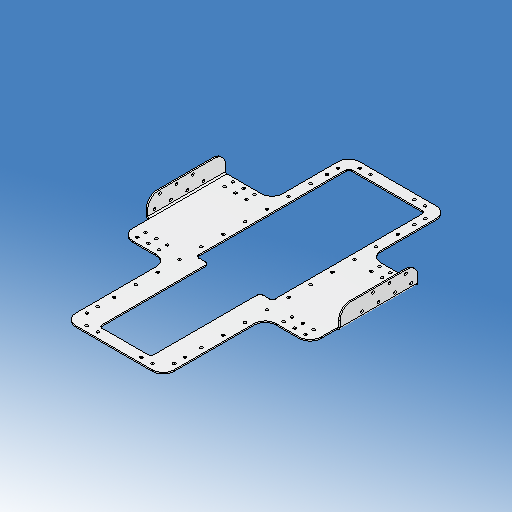
# Autodesk Inventor part: Centerpiece_bottomPlate
Saved by Autodesk Inventor 2025 (Build 290162000, 162)
## iProperties
Created: 2022-10-10
Part Number: Centerpiece_bottomPlate
Material: Aluminum 6061
Document SubType Name: Sheet Metal
Designer: Nebil
Density: 2.7 g/cm^3
Appearance: Aluminum - Flat
Sheet Metal Rule: Default
Author: Nebil
Autodesk Inventor part; units mm, degrees
ref_plane "YZ Plane" through (0, 0, 0) normal (1, 0, 0) x (0, 1, 0)
ref_plane "XZ Plane" through (0, 0, 0) normal (0, 1, 0) x (-1, 0, 0)
ref_plane "XY Plane" through (0, 0, 0) normal (0, 0, 1) x (1, 0, 0)
sketch "Sketch1" plane through (0, 0, 0) normal (0, 1, 0) x (-1, 0, 0)
  line L0 (-114.3, -330.2) -> (114.3, -330.2)
  line L1 (114.3, -330.2) -> (114.3, 330.2)
  line L2 (114.3, 330.2) -> (-114.3, 330.2)
  line L3 (-114.3, 330.2) -> (-114.3, -330.2)
  line L4 (-114.3, -330.2) -> (114.3, 330.2) construction
  line L5 (114.3, -330.2) -> (-114.3, 330.2) construction
  point P0 (0, 0)
  dimension "d0" = 228.6
  dimension "d1" = 660.4
  constraints: 12 end point, 2 midpoint, 2 parallel, 1 horizontal, 1 perpendicular
  measures "d0" distance of L2.end L1.end
  measures "d1" distance of L1.end L0.end
extrude "Extrusion1" add sketch "Sketch1" along normal blind 3.175
sketch "Sketch2" plane through (0, 3.175, 0) normal (0, 1, 0) x (1, 0, 0)
  line L0 (-114.3, 330.2) -> (-114.3, -330.2) construction
  line L1 (-114.3, -304.8) -> (114.3, -304.8) construction
  line L2 (114.3, -330.2) -> (114.3, 330.2) construction
  line L3 (-114.3, -330.2) -> (114.3, -330.2) construction
  line L4 (-114.3, 304.8) -> (114.3, 304.8) construction
  line L5 (114.3, 330.2) -> (-114.3, 330.2) construction
  line L6 (88.9, 330.2) -> (88.9, -344.7266) construction
  line L7 (-88.9, 330.2) -> (-88.9, -330.2) construction
  circle A0 centre (101.6, -292.1) radius 3.175
  line L8 (-114.3, 0) -> (114.3, 0) construction
  circle A1 centre (76.2, -317.5) radius 3.175
  line L9 (0, 330.2) -> (0, -330.2) construction
  point P0 (0, 0)
  dimension "d4" = 25.4
  dimension "d5" = 25.4
  dimension "d6" = 25.4
  dimension "d7" = 25.4
  dimension "d8" = 6.35
  dimension "d9" = 12.7
  dimension "d10" = 12.7
  dimension "d11" = 6.35
  dimension "d12" = 12.7
  dimension "d13" = 12.7
  constraints: 12 end point, 7 point on line, 4 midpoint, 3 perpendicular, 2 centre point, 1 horizontal
  measures "d4" distance between parallel lines of L3 L1
  measures "d5" distance between parallel lines of L4 L5
  measures "d6" distance between parallel lines of L2 L6
  measures "d7" distance between parallel lines of L0 L7
  measures "d8" diameter of A0
  measures "d9" distance from line of A0.centre L6
  measures "d10" distance from line of L1 A0.centre
  measures "d11" diameter of A1
  measures "d12" distance from line of A1.centre L1
  measures "d13" distance from line of L6 A1.centre
extrude "Extrusion2" cut sketch "Sketch2" against normal through all contours A1
extrude "Extrusion3" cut sketch "Sketch2" against normal blind 25.4 contours A0
pattern_linear "Rectangular Pattern3" count 2 spacing 25.4 along (-1, 0, 0) of "Extrusion2"
pattern_linear "Rectangular Pattern2" count 2 spacing 25.4 along (0, 0, -1) of "Extrusion3"
mirror "Mirror2" about plane through (0, 0, 0) normal (1, 0, 0) of "Extrusion3", "Rectangular Pattern2", "Extrusion2", "Rectangular Pattern3"
sketch "Sketch3" plane through (0, 3.175, 0) normal (0, 1, 0) x (1, 0, 0)
  circle A0 centre (101.6, -266.7) radius 3.175 projected
  circle A1 centre (101.6, -228.6) radius 3.175
  line L0 (114.3, -330.2) -> (114.3, 330.2) projected
  circle A2 centre (101.6, -177.8) radius 3.175
  circle A3 centre (101.6, -127) radius 3.175
  circle A4 centre (101.6, -76.2) radius 3.175
  circle A5 centre (101.6, -25.4) radius 3.175
  circle A6 centre (101.6, 25.4) radius 3.175
  circle A7 centre (101.6, 76.2) radius 3.175
  circle A8 centre (101.6, 127) radius 3.175
  circle A9 centre (101.6, 177.8) radius 3.175
  circle A10 centre (101.6, 228.6) radius 3.175
  point P0 (0, 0)
  dimension "d24" = 6.35
  dimension "d25" = 6.35
  dimension "d26" = 38.1
  dimension "d29" = 50.8
  constraints: 10 centre point, 1 vertical, 1 vertical alignment, 18 other
  measures "d24" diameter of A0
  measures "d25" diameter of A1
  measures "d26" distance of A0.centre A1.centre
  measures "d29" distance of A1.centre A2.centre
extrude "Extrusion4" cut sketch "Sketch3" against normal blind 25.4 contours A1 | A2 | A3 | A4 | A5 | A6 | A7 | A8 | A9 | A10
mirror "Mirror3" about plane through (0, 0, 0) normal (1, 0, 0) of "Extrusion4"
mirror "Mirror4" about plane through (0, 0, 0) normal (0, 0, 1) of "Rectangular Pattern3", "Rectangular Pattern2", "Extrusion3", "Extrusion2", "Mirror2"
sketch "Sketch4" plane through (0, 3.175, 0) normal (0, 1, 0) x (1, 0, 0)
  line L0 (-114.3, -151.384) -> (-225.425, -151.384)
  line L1 (-225.425, -151.384) -> (-225.425, 29.591)
  line L2 (-225.425, 29.591) -> (-114.3, 29.591)
  line L3 (-114.3, 29.591) -> (-114.3, -151.384)
  line L4 (-114.3, -330.2) -> (114.3, -330.2) projected
  line L5 (114.3, 330.2) -> (-114.3, 330.2) projected
  line L6 (0, -330.2) -> (0, 330.2) construction
  line L7 (-114.3, 330.2) -> (-114.3, -330.2) construction
  line L8 (114.3, -330.2) -> (114.3, 330.2) projected
  line L9 (114.3, -151.384) -> (225.425, -151.384)
  line L10 (225.425, -151.384) -> (225.425, 29.591)
  line L11 (225.425, 29.591) -> (114.3, 29.591)
  line L12 (114.3, 29.591) -> (114.3, -151.384)
  line L13 (-225.425, 29.591) -> (-114.3, 29.591)
  line L14 (-114.3, 29.591) -> (-114.3, 93.091)
  line L15 (-114.3, 93.091) -> (-219.075, 93.091)
  line L16 (-219.075, 93.091) -> (-219.075, 29.591)
  line L17 (225.425, 29.591) -> (114.3, 29.591)
  line L18 (114.3, 29.591) -> (114.3, 93.091)
  line L19 (114.3, 93.091) -> (219.075, 93.091)
  line L20 (219.075, 93.091) -> (219.075, 29.591)
  line L21 (-95.4828, -304.8) -> (88.9, -304.8) construction
  line L22 (88.9, -304.8) -> (88.9, 304.8) construction
  line L23 (88.9, 304.8) -> (-88.9, 304.8) construction
  line L24 (-88.9, 304.8) -> (-88.9, -304.8) construction
  circle A0 centre (-195.8977, 80.391) radius 3.175
  circle A1 centre (-170.4977, 80.391) radius 3.175
  circle A2 centre (-145.0977, 80.391) radius 3.175
  circle A3 centre (-195.8977, 61.341) radius 3.175
  circle A4 centre (-170.4977, 61.341) radius 3.175
  circle A5 centre (-145.0977, 61.341) radius 3.175
  circle A6 centre (-195.8977, -141.859) radius 3.175
  circle A7 centre (-170.4977, -141.859) radius 3.175
  circle A8 centre (-145.0977, -141.859) radius 3.175
  circle A9 centre (-195.8977, -122.809) radius 3.175
  circle A10 centre (-170.4977, -122.809) radius 3.175
  circle A11 centre (-145.0977, -122.809) radius 3.175
  circle A12 centre (195.8977, 80.391) radius 3.175
  circle A13 centre (170.4977, 80.391) radius 3.175
  circle A14 centre (145.0977, 80.391) radius 3.175
  circle A15 centre (195.8977, 61.341) radius 3.175
  circle A16 centre (170.4977, 61.341) radius 3.175
  circle A17 centre (145.0977, 61.341) radius 3.175
  circle A18 centre (195.8977, -141.859) radius 3.175
  circle A19 centre (170.4977, -141.859) radius 3.175
  circle A20 centre (145.0977, -141.859) radius 3.175
  circle A21 centre (195.8977, -122.809) radius 3.175
  circle A22 centre (170.4977, -122.809) radius 3.175
  circle A23 centre (145.0977, -122.809) radius 3.175
  line L25 (-88.9, 304.8) -> (-60.325, 304.8) construction
  line L26 (-60.325, 304.8) -> (-60.325, 50.8)
  line L27 (-60.325, 50.8) -> (-88.9, 50.8)
  line L28 (-88.9, 50.8) -> (-88.9, 304.8) construction
  line L29 (88.9, 304.8) -> (60.325, 304.8) construction
  line L30 (60.325, 304.8) -> (60.325, 50.8)
  line L31 (60.325, 50.8) -> (88.9, 50.8)
  line L32 (88.9, 50.8) -> (88.9, 304.8) construction
  line L33 (-88.9, -304.8) -> (-88.9, 50.8)
  line L34 (88.9, -304.8) -> (88.9, 50.8)
  line L35 (-88.9, -304.8) -> (88.9, -304.8)
  line L36 (-60.325, 304.8) -> (60.325, 304.8)
  point P0 (0, 0)
  point P1 (114.3, -151.384)
  point P2 (114.3, 29.591)
  point P3 (114.3, 29.591)
  dimension "d39" = 111.125
  dimension "d40" = 178.816
  dimension "d88" = 180.975
  dimension "d90" = 25.4
  dimension "d91" = 25.4
  dimension "d92" = 25.4
  dimension "d94" = 6.35
  dimension "d97" = 25.4
  dimension "d100" = 19.05
  dimension "d103" = 231.775
  dimension "d108" = 6.35
  dimension "d109" = 6.35
  dimension "d110" = 81.5977
  dimension "d111" = 6.35
  dimension "d114" = 25.4
  dimension "d117" = 19.05
  dimension "d122" = 9.525
  dimension "d123" = 25.4
  dimension "d124" = 254
  dimension "d125" = 28.575
  constraints: 66 end point, 24 centre point, 14 symmetric about line, 12 parallel, 8 horizontal, 8 perpendicular, 7 point on line, 5 collinear, 4 equal length, 2 midpoint, 2 vertical, 1 vertical alignment, 32 other
  measures "d39" distance between parallel lines of L3 L1
  measures "d40" distance between parallel lines of L0 L4
  measures "d88" distance of L0.end L1.end
  measures "d90" distance between parallel lines of L23 L5
  measures "d91" distance between parallel lines of L8 L22
  measures "d92" distance between parallel lines of L7 L24
  measures "d94" diameter of A0
  measures "d97" distance of A0.centre A1.centre
  measures "d100" distance of A0.centre A3.centre
  measures "d103" distance from line of L0 A0.centre
  measures "d108" distance between parallel lines of L16 L1
  measures "d109" distance between parallel lines of L10 L20
  measures "d110" distance from line of L7 A0.centre
  measures "d111" diameter of A6
  measures "d114" distance of A6.centre A7.centre
  measures "d117" distance of A6.centre A9.centre
  measures "d122" distance from line of L0 A6.centre
  measures "d123" distance between parallel lines of L21 L4
  measures "d124" distance between parallel lines of L25 L27
  measures "d125" distance of L26.end L27.end
extrude "Extrusion5" add sketch "Sketch4" against normal up to surface (3.175 mm away) contours L0 L1 L2 L3 | L8 L11 L10 L9 | A6 | A7 | A8 | A9 | A10 | A11 | A18 | A19 | A20 | A21 | A22 | A23
sketch "Sketch5" plane through (-222.25, 3.175, 151.384) normal (-1, 0, 0) x (0, 1, 0)
  line L0 (0, -180.975) -> (0, 0)
  line L1 (0, 0) -> (-45.8301, 0)
  line L2 (-45.8301, 0) -> (-45.8301, -180.975)
  line L3 (-45.8301, -180.975) -> (0, -180.975)
  constraints: 6 end point, 1 horizontal, 1 perpendicular, 1 vertical
edge flange "Flange1" height 45.8301 angle 90 thickness 3.175 bend radius 3.175 thickness toward (-1, 0, 0) relief tear relief width 3.175 relief depth 1.5875 corner gap 3.175 corner form 0 edges at (-225.425, 3.175, 60.8965) (225.425, 3.175, 60.8965) wall of the first edge with corners at (-222.25, 3.175, -29.591) (-222.25, 3.175, 151.384) (-222.25, -42.6551, 151.384) (-222.25, -42.6551, -29.591)
bend "Bend1"
corner "Corner1"
sketch "Sketch6" plane through (225.425, -42.6551, 151.384) normal (1, 0, 0) x (0, 0, -1)
  circle A0 centre (129.999, 32.8083) radius 3.175
  circle A1 centre (104.599, 7.4083) radius 3.175
  line L0 (0, 0) -> (180.975, 0) projected
  circle A2 centre (91.899, 32.8083) radius 3.175
  circle A3 centre (66.499, 7.4083) radius 3.175
  circle A4 centre (53.799, 32.8083) radius 3.175
  circle A5 centre (28.399, 7.4083) radius 3.175
  circle A6 centre (15.699, 32.8083) radius 3.175
  line L1 (180.975, 39.4801) -> (180.975, 0) projected
  point P0 (151.384, 42.6551)
  dimension "d56" = 6.35
  dimension "d57" = 25.4
  dimension "d58" = 25.4
  dimension "d61" = 38.1
  dimension "d66" = 38.1
  dimension "d67" = 7.4083
  dimension "d86" = 50.976
  constraints: 7 centre point, 2 equal radius, 1 horizontal, 1 horizontal alignment, 8 other
  measures "d56" diameter of A0
  measures "d57" horizontal distance of A1.centre A0.centre
  measures "d58" horizontal distance of A1.centre A0.centre
  measures "d61" distance of A0.centre A2.centre
  measures "d66" distance of A6.centre A4.centre
  measures "d67" distance from line of A1.centre L0
  measures "d86" distance from line of A0.centre L1
extrude "Cut1" cut sketch "Sketch6" against normal blind 3.175
sketch "Sketch7" plane through (-225.425, -42.6551, -29.591) normal (-1, 0, 0) x (0, 0, 1)
  circle A0 centre (129.999, 32.8083) radius 3.175
  circle A1 centre (104.599, 7.4083) radius 3.175
  line L0 (0, 0) -> (180.975, 0) projected
  line L1 (180.975, 39.4801) -> (180.975, 0) projected
  circle A2 centre (91.899, 32.8083) radius 3.175
  circle A3 centre (66.499, 7.4083) radius 3.175
  circle A4 centre (53.799, 32.8083) radius 3.175
  circle A5 centre (28.399, 7.4083) radius 3.175
  circle A6 centre (15.699, 32.8083) radius 3.175
  point P0 (29.591, 42.6551)
  dimension "d70" = 6.35
  dimension "d71" = 6.35
  dimension "d72" = 25.4
  dimension "d73" = 25.4
  dimension "d74" = 7.4083
  dimension "d75" = 50.976
  dimension "d78" = 38.1
  dimension "d83" = 6.35
  dimension "d87" = 38.1
  constraints: 7 centre point, 1 horizontal, 1 horizontal alignment, 8 other
  measures "d70" diameter of A0
  measures "d71" diameter of A1
  measures "d72" horizontal distance of A1.centre A0.centre
  measures "d73" horizontal distance of A1.centre A0.centre
  measures "d74" distance from line of L0 A1.centre
  measures "d75" distance from line of A0.centre L1
  measures "d78" distance of A0.centre A2.centre
  measures "d83" diameter of A6
  measures "d87" distance of A6.centre A4.centre
extrude "Cut2" cut sketch "Sketch7" against normal blind 3.175
extrude "Extrusion6" add sketch "Sketch4" against normal up to surface (3.175 mm away) contours L2 L16 L15 L14 | L8 L19 L20 L11
fillet "Fillet1" radius 25.4 14 edges at (-219.075, 1.5875, -93.091) (219.075, 1.5875, -93.091) (-114.3, 1.5875, -93.091) (114.3, 1.5875, -93.091) (114.3, 1.5875, 151.384) (-114.3, 1.5875, 151.384) (114.3, 1.5875, -330.2) (-114.3, 1.5875, -330.2) (114.3, 1.5875, 330.2) (-114.3, 1.5875, 330.2) (223.8375, -42.6551, -29.591) (-223.8375, -42.6551, -29.591) (223.8375, -42.6551, 151.384) (-223.8375, -42.6551, 151.384)
extrude "Extrusion7" cut sketch "Sketch4" against normal blind 25.4 contours A6 | A7 | A8 | A9 | A10 | A11 | A18 | A19 | A20 | A21 | A22 | A23 | L36 L30 L31 L34 L35 L33 L27 L26
fillet "Fillet2" radius 6.35 8 edges at (60.325, 1.5875, -50.8) (-60.325, 1.5875, -50.8) (-88.9, 1.5875, -50.8) (-60.325, 1.5875, -304.8) (60.325, 1.5875, -304.8) (88.9, 1.5875, -50.8) (88.9, 1.5875, 304.8) (-88.9, 1.5875, 304.8)
equation "\"d25\" = d24"
equation "\"d68\" = Thickness"
equation "\"d84\" = Thickness"
equation "\"d44\" = Thickness"
equation "\"d45\" = BendReliefWidth"
equation "\"d46\" = BendReliefDepth"
equation "\"d47\" = MinimumRemnant"
equation "\"d48\" = TransitionRadius"
equation "\"d51\" = BendRadius"
equation "\"d52\" = CornerReliefSize"
equation "\"d53\" = GapSize"
equation "\"d54\" = JacobiRadiusSize"
equation "\"BendRadius\" = Thickness"
equation "\"BendReliefWidth\" = Thickness"
equation "\"BendReliefDepth\" = 0.5 * Thickness"
equation "\"CornerReliefSize\" = 4 * Thickness"
equation "\"MinimumRemnant\" = 2 * Thickness"
equation "\"TransitionRadius\" = BendRadius"
equation "\"JacobiRadiusSize\" = BendRadius"
equation "\"GapSize\" = Thickness"
equation "\"Thickness\" = 3.175"
body "Solid1"
